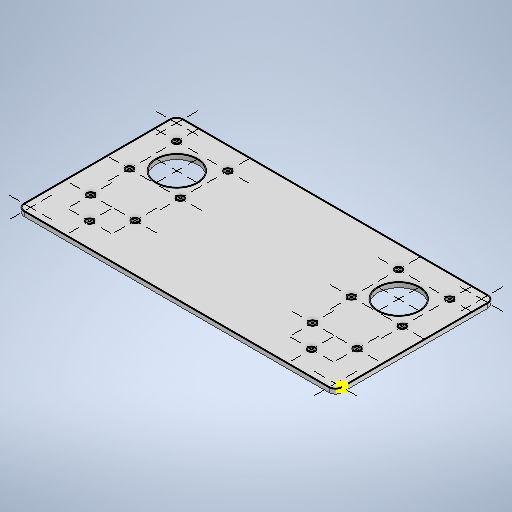
# Autodesk Inventor part: body_bottom_frame
Saved by Autodesk Inventor 2026.1 (Build 301233000, 233)
## iProperties
Created: 2025-08-16
Part Number: body_bottom_frame
Material: Generic
Document SubType Name: Modeling
Designer: chris
Density: 1 g/cm^3
Appearance: Default
Author: chris
Autodesk Inventor part; units mm, degrees
ref_plane "YZ Plane" through (0, 0, 0) normal (1, 0, 0) x (0, 1, 0)
ref_plane "XZ Plane" through (0, 0, 0) normal (0, 1, 0) x (-1, 0, 0)
ref_plane "XY Plane" through (0, 0, 0) normal (0, 0, 1) x (1, 0, 0)
sketch "Sketch1" plane through (0, 0, 0) normal (0, 1, 0) x (-1, 0, 0)
  circle A0 centre (15.07, -33) radius 6.5
  circle A1 centre (84.93, -33) radius 6.5
  circle A2 centre (15.07, -5.58) radius 1.05
  circle A3 centre (22.07, -12.88) radius 1.05
  circle A4 centre (8.07, -12.88) radius 1.05
  circle A5 centre (23.07, -26.1) radius 1.05
  circle A6 centre (7.07, -26.1) radius 1.05
  circle A7 centre (7, -41) radius 1.05
  circle A8 centre (23.14, -41) radius 1.05
  circle A9 centre (93, -41) radius 1.05
  circle A10 centre (76.86, -41) radius 1.05
  circle A11 centre (76.93, -26.1) radius 1.05
  circle A12 centre (92.93, -26.1) radius 1.05
  circle A13 centre (91.93, -12.88) radius 1.05
  circle A14 centre (77.93, -12.88) radius 1.05
  circle A15 centre (84.93, -5.58) radius 1.05
  arc A16 (100, 0) -> (98, 2) centre (98, 0) ccw
  line L0 (100, 0) -> (100, -46)
  line L1 (2, 2) -> (98, 2)
  arc A17 (2, 2) -> (0, 0) centre (2, 0) ccw
  line L2 (0, -46) -> (0, 0)
  arc A18 (0, -46) -> (2, -48) centre (2, -46) ccw
  line L3 (98, -48) -> (2, -48)
  arc A19 (98, -48) -> (100, -46) centre (98, -46) ccw
  point P0 (0, 0)
  constraints: 20 centre point, 17 equal radius, 8 end point, 8 point on circle, 8 tangent, 2 horizontal, 2 perpendicular, 2 vertical, 1 parallel, 49 other
extrude "Extrusion1" add sketch "Sketch1" against normal blind 1.5
body "Solid1"
